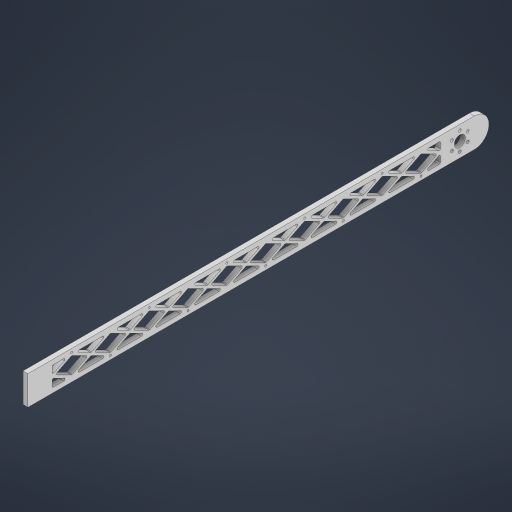
# Autodesk Inventor part: Arm
Saved by Autodesk Inventor 2023 (Build 270158000, 158)
## iProperties
Created: 2023-01-21
Part Number: Arm
Material: Generic
Document SubType Name: Modeling
Designer: Terrence
Density: 1 g/cm^3
Appearance: Default
Author: Terrence
Autodesk Inventor part; units mm, degrees
ref_plane "YZ Plane" through (0, 0, 0) normal (1, 0, 0) x (0, 1, 0)
ref_plane "XZ Plane" through (0, 0, 0) normal (0, 1, 0) x (-1, 0, 0)
ref_plane "XY Plane" through (0, 0, 0) normal (0, 0, 1) x (1, 0, 0)
sketch "Sketch1" plane through (0, 0, 0) normal (1, 0, 0) x (0, 1, 0)
  line L0 (0, 0) -> (76.2, 0)
  line L1 (76.2, 0) -> (76.2, -1193.8)
  line L2 (76.2, -1193.8) -> (0, -1193.8)
  line L3 (0, -1193.8) -> (0, 0)
  dimension "d0" = 76.2
  dimension "d1" = 1193.8
  constraints: 8 end point, 2 parallel, 1 horizontal, 1 perpendicular
  measures "d0" distance of L1.end L2.end
  measures "d1" distance of L0.end L1.end
extrude "Extrusion1" add sketch "Sketch1" along normal blind 12.7
sketch "Sketch2" plane through (12.7, 0, 0) normal (1, 0, 0) x (0, 0, -1)
  line L0 (1193.8, 76.2) -> (0, 76.2) projected
  line L1 (1117.6, 76.2) -> (1117.6, 0) construction
  line L2 (0, 0) -> (1193.8, 0) projected
  circle A0 centre (1117.6, 38.1) radius 14.2875
  dimension "d5" = 1117.6
  dimension "d24" = 28.575
  constraints: 2 end point, 2 point on line, 1 centre point, 1 midpoint, 1 perpendicular
  measures "d5" distance from line of L2.start L1
  measures "d24" diameter of A0
extrude "Extrusion2" cut sketch "Sketch2" against normal through all
fillet "Fillet1" radius 38.1 2 edges at (6.35, 76.2, -1193.8) (6.35, 0, -1193.8)
sketch "Sketch3" plane through (12.7, 0, 0) normal (1, 0, 0) x (0, 0, -1)
  line L0 (50.8, 63.5) -> (1066.8, 63.5)
  line L1 (1066.8, 63.5) -> (1066.8, 12.7)
  line L2 (1066.8, 12.7) -> (50.8, 12.7)
  line L3 (50.8, 12.7) -> (50.8, 63.5)
  line L4 (0, 0) -> (1155.7, 0) projected
  line L5 (1155.7, 76.2) -> (0, 76.2) projected
  line L6 (0, 76.2) -> (0, 0) projected
  dimension "d9" = 12.7
  dimension "d10" = 12.7
  dimension "d11" = 50.8
  dimension "d12" = 1016
  constraints: 8 end point, 2 parallel, 1 horizontal, 1 perpendicular
  measures "d9" distance between parallel lines of L4 L2
  measures "d10" distance between parallel lines of L5 L0
  measures "d11" distance between parallel lines of L6 L3
  measures "d12" distance of L1.end L2.end
extrude "Extrusion3" cut sketch "Sketch3" against normal through all
sketch "Sketch4" plane through (12.7, 0, 0) normal (1, 0, 0) x (0, 0, -1)
  line L0 (50.8, 63.5) -> (152.4, 63.5) construction
  line L1 (152.4, 63.5) -> (152.4, 12.7) construction
  line L2 (152.4, 12.7) -> (50.8, 12.7) construction
  line L3 (50.8, 12.7) -> (50.8, 63.5) construction
  line L4 (50.8, 38.1) -> (101.6, 63.5) construction
  line L5 (101.6, 63.5) -> (152.4, 38.1) construction
  line L6 (152.4, 38.1) -> (101.6, 12.7) construction
  line L7 (101.6, 12.7) -> (50.8, 38.1) construction
  line L8 (49.3801, 40.9398) -> (100.1801, 66.3398)
  line L9 (100.1801, 66.3398) -> (103.0199, 60.6602)
  line L10 (103.0199, 60.6602) -> (52.2199, 35.2602)
  line L11 (52.2199, 35.2602) -> (49.3801, 40.9398)
  line L12 (49.3801, 40.9398) -> (103.0199, 60.6602) construction
  line L13 (100.1801, 66.3398) -> (52.2199, 35.2602) construction
  line L14 (153.8199, 40.9398) -> (103.0199, 66.3398)
  line L15 (103.0199, 66.3398) -> (100.1801, 60.6602)
  line L16 (100.1801, 60.6602) -> (150.9801, 35.2602)
  line L17 (150.9801, 35.2602) -> (153.8199, 40.9398)
  line L18 (153.8199, 40.9398) -> (100.1801, 60.6602) construction
  line L19 (103.0199, 66.3398) -> (150.9801, 35.2602) construction
  line L20 (49.3801, 35.2602) -> (100.1801, 9.8602)
  line L21 (100.1801, 9.8602) -> (103.0199, 15.5398)
  line L22 (103.0199, 15.5398) -> (52.2199, 40.9398)
  line L23 (52.2199, 40.9398) -> (49.3801, 35.2602)
  line L24 (49.3801, 35.2602) -> (103.0199, 15.5398) construction
  line L25 (100.1801, 9.8602) -> (52.2199, 40.9398) construction
  line L26 (100.1801, 15.5398) -> (150.9801, 40.9398)
  line L27 (150.9801, 40.9398) -> (153.8199, 35.2602)
  line L28 (153.8199, 35.2602) -> (103.0199, 9.8602)
  line L29 (103.0199, 9.8602) -> (100.1801, 15.5398)
  line L30 (100.1801, 15.5398) -> (153.8199, 35.2602) construction
  line L31 (150.9801, 40.9398) -> (103.0199, 9.8602) construction
  point P0 (0, 0)
  point P1 (50.8, 12.7)
  point P2 (76.2, 50.8)
  point P3 (127, 50.8)
  point P4 (76.2, 25.4)
  point P5 (127, 25.4)
  point P6 (50.8, 38.1)
  point P7 (101.6, 12.7)
  point P8 (101.6, 59.9502)
  point P9 (145.3005, 38.1)
  point P10 (101.6, 16.2498)
  point P11 (57.8995, 38.1)
  point P12 (101.6, 63.5)
  point P13 (152.4, 38.1)
  dimension "d15" = 101.6
  dimension "d16" = 6.35
  dimension "d17" = 6.35
  constraints: 64 end point, 22 midpoint, 13 parallel, 5 perpendicular, 2 coincident, 2 equal length, 1 horizontal
  measures "d15" distance of L1.end L2.end
  measures "d16" distance of L8.end L9.end
  measures "d17" distance of L15.end L14.end
extrude "Extrusion4" add sketch "Sketch4" against normal up to surface (12.7 mm away) contours L8 L9 L15 L16 L10 L22 L23 L11 | L23 L22 L10 L11 | L11 L10 L22 L26 L29 L21 L20 L23 | L15 L14 L17 L27 L26 L16 L10 L9 | L9 L10 L16 L15 | L26 L16 L17 L27 L28 L29 L21 L22 | L22 L21 L29 L26 | L26 L27 L17 L16
pattern_linear "Rectangular Pattern1" count 10 spacing 101.6 along (0, 0, -1) of "Extrusion4"
fillet "Fillet2" radius 3.175 106 edges at (6.35, 12.7, -50.8) (6.35, 34.5502, -50.8) (6.35, 12.7, -94.5005) (6.35, 16.2498, -101.6) (6.35, 38.1, -57.8995) (6.35, 38.1, -145.3005) (6.35, 59.9502, -101.6) (6.35, 12.7, -196.1005) (6.35, 12.7, -108.6995) (6.35, 12.7, -297.7005) (6.35, 12.7, -210.2995) (6.35, 12.7, -399.3005) (6.35, 12.7, -311.8995) (6.35, 12.7, -500.9005) (6.35, 12.7, -413.4995) (6.35, 12.7, -602.5005) (6.35, 12.7, -515.0995) (6.35, 12.7, -704.1005) (6.35, 12.7, -616.6995) (6.35, 12.7, -805.7005) (6.35, 12.7, -718.2995) (6.35, 12.7, -907.3005) (6.35, 12.7, -819.8995) (6.35, 12.7, -1008.9005) (6.35, 12.7, -921.4995) (6.35, 12.7, -1066.8) (6.35, 12.7, -1023.0995) (6.35, 34.5502, -1066.8) (6.35, 63.5, -1066.8) (6.35, 41.6498, -1066.8) (6.35, 63.5, -1023.0995) (6.35, 63.5, -921.4995) (6.35, 63.5, -1008.9005) (6.35, 63.5, -819.8995) (6.35, 63.5, -907.3005) (6.35, 63.5, -718.2995) (6.35, 63.5, -805.7005) (6.35, 63.5, -616.6995) (6.35, 63.5, -704.1005) (6.35, 63.5, -515.0995) (6.35, 63.5, -602.5005) (6.35, 63.5, -413.4995) (6.35, 63.5, -500.9005) (6.35, 63.5, -311.8995) (6.35, 63.5, -399.3005) (6.35, 63.5, -210.2995) (6.35, 63.5, -297.7005) (6.35, 63.5, -108.6995) (6.35, 63.5, -196.1005) (6.35, 41.6498, -152.4) (6.35, 34.5502, -152.4) (6.35, 41.6498, -50.8) (6.35, 63.5, -50.8) (6.35, 63.5, -94.5005) (6.35, 41.6498, -254) (6.35, 34.5502, -254) (6.35, 59.9502, -203.2) (6.35, 38.1, -246.9005) (6.35, 38.1, -159.4995) (6.35, 16.2498, -203.2) (6.35, 34.5502, -355.6) (6.35, 34.5502, -457.2) (6.35, 34.5502, -558.8) (6.35, 34.5502, -660.4) (6.35, 34.5502, -762) (6.35, 34.5502, -863.6) (6.35, 34.5502, -965.2) (6.35, 41.6498, -965.2) (6.35, 41.6498, -863.6) (6.35, 41.6498, -762) (6.35, 41.6498, -660.4) (6.35, 41.6498, -558.8) (6.35, 41.6498, -457.2) (6.35, 41.6498, -355.6) (6.35, 59.9502, -304.8) (6.35, 38.1, -348.5005) (6.35, 38.1, -261.0995) (6.35, 16.2498, -304.8) (6.35, 59.9502, -406.4) (6.35, 38.1, -450.1005) (6.35, 38.1, -362.6995) (6.35, 16.2498, -406.4) (6.35, 59.9502, -508) (6.35, 38.1, -551.7005) (6.35, 38.1, -464.2995) (6.35, 16.2498, -508) (6.35, 59.9502, -609.6) (6.35, 38.1, -653.3005) (6.35, 38.1, -565.8995) (6.35, 16.2498, -609.6) (6.35, 59.9502, -711.2) (6.35, 38.1, -754.9005) (6.35, 38.1, -667.4995) (6.35, 16.2498, -711.2) (6.35, 59.9502, -812.8) (6.35, 38.1, -856.5005) (6.35, 38.1, -769.0995) (6.35, 16.2498, -812.8) (6.35, 59.9502, -914.4) (6.35, 38.1, -958.1005) (6.35, 38.1, -870.6995) (6.35, 16.2498, -914.4) (6.35, 59.9502, -1016) (6.35, 38.1, -1059.7005) (6.35, 38.1, -972.2995) (6.35, 16.2498, -1016)
sketch "Sketch5" plane through (12.7, 0, 0) normal (1, 0, 0) x (0, 0, -1)
  circle A0 centre (1117.6, 38.1) radius 14.2875 projected
  line L0 (1117.6, 38.1) -> (1117.6, 61.9252) construction
  circle A1 centre (1117.6, 61.9252) radius 3.6233
  point P0 (0, 0)
  dimension "d32" = 23.8252
  constraints: 2 end point, 1 centre point, 1 coincident, 1 vertical
  measures "d32" distance of L0.start L0.end
extrude "Extrusion5" cut sketch "Sketch5" against normal through all contours A1
pattern_circular "Circular Pattern1" count 6 over 360 about axis through (12.7, 38.1, -1117.6) along (-1, 0, 0) of "Extrusion5"
sketch "Sketch6" plane through (12.7, 0, 0) normal (1, 0, 0) x (0, 0, -1)
  circle A0 centre (101.6, 66.675) radius 2.54
  arc A1 (103.0199, 59.2403) -> (100.1801, 59.2403) centre (101.6, 56.4005) ccw projected
  line L0 (101.6, 59.5755) -> (101.6, 76.2) construction
  line L1 (1155.7, 76.2) -> (0, 76.2) projected
  line L2 (101.6, 56.4005) -> (101.6, 58.6744) construction
  circle A2 centre (203.2, 9.525) radius 2.54
  arc A3 (201.7801, 16.9597) -> (204.6199, 16.9597) centre (203.2, 19.7995) ccw projected
  line L3 (203.2, 19.7995) -> (203.2, 16.6245)
  line L4 (0, 0) -> (1155.7, 0) projected
  dimension "d33" = 9.525
  dimension "d34" = 5.08
  dimension "d35" = 9.525
  dimension "d36" = 5.08
  constraints: 6 end point, 3 point on line, 3 vertical, 2 centre point, 2 point on circle, 1 collinear
  measures "d33" distance of L0.end A0.centre
  measures "d34" diameter of A0
  measures "d35" distance from line of L4 A2.centre
  measures "d36" diameter of A2
extrude "Extrusion6" cut sketch "Sketch6" against normal blind 25.4
pattern_linear "Rectangular Pattern2" count 5 spacing -203.2 along (0, 0, 1) of "Extrusion6"
sketch "Sketch7" plane through (0, 0, 0) normal (0, 0, 1) x (1, 0, 0)
  line L0 (0, 0) -> (0, 76.2) projected
  line L1 (0, 76.2) -> (12.7, 76.2) projected
  line L2 (12.7, 76.2) -> (12.7, 0) projected
  line L3 (12.7, 0) -> (0, 0) projected
extrude "Extrusion7" add sketch "Sketch7" along normal blind 12.7
body "Solid1"
